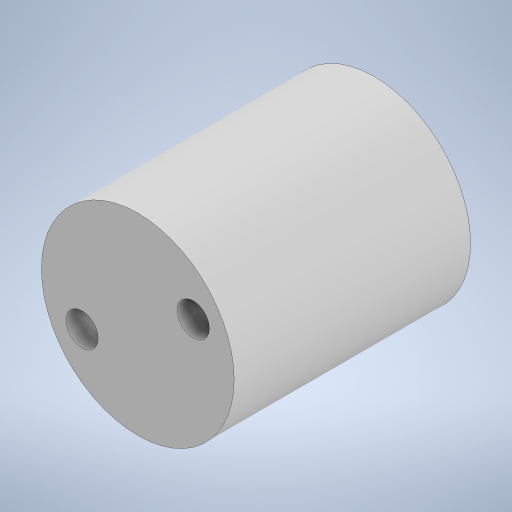
# Autodesk Inventor part: Crankshaft
Saved by Autodesk Inventor 2023 (Build 270158000, 158)
## iProperties
Created: 2022-10-29
Part Number: Crankshaft
Material: Generic
Document SubType Name: Modeling
Designer: tommy
Density: 1 g/cm^3
Appearance: Default
Author: tommy
Autodesk Inventor part; units mm, degrees
ref_plane "YZ Plane" through (0, 0, 0) normal (1, 0, 0) x (0, 1, 0)
ref_plane "XZ Plane" through (0, 0, 0) normal (0, 1, 0) x (-1, 0, 0)
ref_plane "XY Plane" through (0, 0, 0) normal (0, 0, 1) x (1, 0, 0)
sketch "Sketch1" plane through (0, 0, 0) normal (0, 0, 1) x (1, 0, 0)
  circle A0 centre (0, 0) radius 9.525
  circle A1 centre (0, -6.35) radius 1.5875
  circle A2 centre (0, 6.35) radius 1.5875
  line L0 (0, 9.525) -> (0, -9.525)
  dimension "d3" = 3.175
  dimension "d4" = 3.175
  constraints: 3 centre point, 2 end point, 2 point on circle, 1 vertical
  measures "d3" diameter of A1
  measures "d4" diameter of A2
extrude "Extrusion2" add sketch "Sketch1" along normal blind 23.368
extrude "Extrusion3" cut sketch "Sketch1" along normal blind 6.35 contours L0 A2 | A2 L0 | L0 A1 | A1 L0
sketch "Sketch2" plane through (0, 0, 23.368) normal (0, 0, 1) x (1, 0, 0)
  circle A0 centre (0, 0) radius 9.525 projected
  line L0 (0, 9.525) -> (0, -9.525)
  line L1 (0, 0) -> (25.4, 0) construction
  line L2 (0, 0) -> (25.4, 0) construction
  line L3 (8.2489, 4.7625) -> (-8.2489, -4.7625)
  line L4 (0, 0) -> (5.4993, 3.175)
  line L5 (5.4993, 3.175) -> (-5.4993, -3.175)
  circle A1 centre (-5.4993, -3.175) radius 1.5875
  circle A2 centre (5.4993, 3.175) radius 1.5875
  line L6 (0, 0) -> (15.1329, 0) construction
  line L7 (8.2489, 4.7625) -> (-8.2489, -4.7625)
  dimension "d22" = 6.35
  dimension "d23" = 12.7
  dimension "d24" = 3.175
  dimension "d25" = 3.175
  constraints: 16 end point, 6 point on circle, 3 horizontal, 2 centre point, 2 coincident, 2 point on line, 1 vertical
  measures "d22" distance of L1.start L4.end
  measures "d23" distance of L4.end L5.end
  measures "d24" diameter of A1
  measures "d25" diameter of A2
extrude "Extrusion4" cut sketch "Sketch2" against normal blind 6.35 contours A2 L3 | L3 A2 | A1 L3 | L3 A1
body "Solid2"
